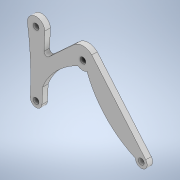
# Autodesk Inventor part: Bracket Concept MK8
Saved by Autodesk Inventor 2021 (Build 250183000, 183)
## iProperties
Created: 2021-05-11
Part Number: Bracket Concept MK8
Material: Generic
Document SubType Name: Modeling
Designer: Jawal
Density: 1 g/cm^3
Appearance: Default
Author: Jawal
Autodesk Inventor part; units mm, degrees
ref_plane "YZ Plane" through (0, 0, 0) normal (1, 0, 0) x (0, 1, 0)
ref_plane "XZ Plane" through (0, 0, 0) normal (0, 1, 0) x (-1, 0, 0)
ref_plane "XY Plane" through (0, 0, 0) normal (0, 0, 1) x (1, 0, 0)
sketch "Sketch1" plane through (0, 0, 0) normal (0, 0, 1) x (1, 0, 0)
  line L0 (-110, 70) -> (110, 70) construction
  line L1 (110, 70) -> (110, -70) construction
  line L2 (110, -70) -> (-110, -70) construction
  line L3 (-110, -70) -> (-110, 70) construction
  circle A0 centre (-90, 55) radius 5
  circle A1 centre (-90, -55) radius 5
  circle A2 centre (90, -55) radius 5
  circle A3 centre (-10, 45) radius 5
  line L4 (-67, 0) -> (-42, 0) construction
  line L5 (-42, 0) -> (-42, -30) construction
  line L6 (-42, -30) -> (-67, -30) construction
  line L7 (-67, -30) -> (-67, 0) construction
  circle A4 centre (-54.5, -19) radius 10 construction
  arc A5 (-75.0363, 56.0433) -> (-104.3936, 50.7781) centre (-90, 55) ccw
  arc A6 (-99.9402, -53.9078) -> (-80.0103, -55.4531) centre (-90, -55) ccw
  arc A7 (-100, -55) -> (-105, 55) centre (-644.4063, -24.6321) ccw
  line L8 (-78.8103, -29) -> (-67, 2.1947) construction
  line L9 (-67, 2.1947) -> (-37.7539, 24.0313) construction
  line L10 (-37.7539, 24.0313) -> (-18.5252, 32.6582) construction
  spline S0 degree 3 poles (-78.8103, -29) (-67, 2.1947) (-37.7539, 24.0313) (-18.5252, 32.6582) knots 1 1 1 1 2 2 2 2
  line L11 (-24.7333, 61.0503) -> (-68.0357, 21.3009)
  line L12 (-75.0363, 56.0433) -> (-76.412, 25.2072)
  line L13 (-78.8103, -29) -> (-80.0103, -55.4531)
  arc A8 (80, -55) -> (97.6312, -48.5374) centre (90, -55) ccw
  line L14 (5.1977, 60.6112) -> (97.6312, -48.5374)
  arc A9 (-2.7947, 31.8439) -> (80, -55) centre (141.6446, 86.6595) ccw
  arc A10 (-18.5252, 32.6582) -> (-2.7947, 31.8439) centre (-10, 45) ccw
  arc A11 (5.1977, 60.6112) -> (-24.7333, 61.0503) centre (-10, 45) ccw
  arc A12 (-76.412, 25.2072) -> (-68.0357, 21.3009) centre (-71.4169, 24.9844) ccw
  point P0 (0, 0)
  dimension "d1" = 70
  dimension "d2" = 70
  dimension "d3" = 110
  dimension "d4" = 110
  dimension "d5" = 10
  dimension "d6" = 10
  dimension "d7" = 10
  dimension "d8" = 10
  dimension "d9" = 55
  dimension "d10" = 55
  dimension "d11" = 55
  dimension "d12" = 180
  dimension "d13" = 90
  dimension "d15" = 10
  dimension "d16" = 45
  dimension "d17" = 42
  dimension "d18" = 30
  dimension "d19" = 0
  dimension "d20" = 25
  dimension "d21" = 20
  dimension "d25" = 19
  dimension "d26" = 12.5
  dimension "d67" = 90
  dimension "d68" = 30
  dimension "d70" = 20
  dimension "d71" = 20
  dimension "d74" = 10
  constraints: 24 end point, 20 point on circle, 13 centre point, 6 tangent, 4 coincident, 4 parallel, 2 horizontal, 2 perpendicular, 1 point on line, 3 other
  measures "d1" distance from line of point (0, 0) L2
  measures "d2" distance from line of point (0, 0) L0
  measures "d3" distance from line of L1 point (0, 0)
  measures "d4" distance from line of point (0, 0) L3
  measures "d5" diameter of A0
  measures "d6" diameter of A1
  measures "d7" diameter of A2
  measures "d8" diameter of A3
  measures "d9" vertical distance of point (0, 0) A0.centre
  measures "d10" vertical distance of point (0, 0) A1.centre
  measures "d11" vertical distance of A2.centre point (0, 0)
  measures "d12" distance of A2.centre A1.centre
  measures "d13" horizontal distance of point (0, 0) A0.centre
  measures "d15" horizontal distance of point (0, 0) A3.centre
  measures "d16" vertical distance of point (0, 0) A3.centre
  measures "d17" distance from line of point (0, 0) L5
  measures "d18" distance of L4.end L5.end
  measures "d19" distance from line of L4 point (0, 0)
  measures "d20" distance of L5.end L6.end
  measures "d21" diameter of A4
  measures "d25" distance from line of L4 A4.centre
  measures "d26" distance from line of L7 A4.centre
  measures "d67" horizontal distance of point (0, 0) A1.centre
  measures "d68" diameter of A5
  measures "d70" diameter of A6
  measures "d71" diameter of A8
  measures "d74" diameter of A12
extrude "Extrusion6" add sketch "Sketch1" along normal blind 9.4 contours L12 A12 L11 A11 L14 A8 A9 A10 S0 L13 A6 A7 A5 | A7 A5
equation "\"d1\" = d2"
equation "\"d4\" = d3"
equation "\"d10\" = d9"
equation "\"d11\" = d9"
equation "\"d26\" = 0.5 * d20"
body "Solid6"
